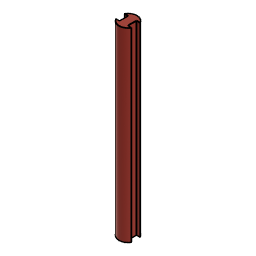
Osa krokoměru v6 (Autodesk Fusion 360 design; units mm, degrees)
Autodesk Fusion 360 part; units mm, degrees
sketch "Profil" plane through (0, 0, 0) normal (0, 0, 1) x (1, 0, 0)
  circle A0 centre (0, 0) radius 4.3
  line L0 (3.8066, -2) -> (-3.8066, -2)
  line L1 (-3.8066, -2) -> (-3.8066, 2)
  line L2 (-3.8066, 2) -> (3.8066, 2)
  line L3 (3.8066, 2) -> (3.8066, -2)
  line L4 (3.8066, -2) -> (-3.8066, 2) construction
  line L5 (-3.8066, -2) -> (3.8066, 2) construction
  line L6 (2, -2) -> (-2, -2)
  line L7 (-2, -2) -> (-2, 2)
  line L8 (-2, 2) -> (2, 2)
  line L9 (2, 2) -> (2, -2)
  line L10 (2, -2) -> (-2, 2) construction
  line L11 (-2, -2) -> (2, 2) construction
  line L12 (3.6946, 2.2) -> (3.6946, -2.2)
  dimension "d1" = 8.6
  dimension "d2" = 4
  dimension "d3" = 4
  dimension "d4" = 0.2
  constraint coincident A0.centre origin
  constraint horizontal L0
  constraint perpendicular L0 L1
  constraint parallel L0 L2
  constraint parallel L1 L3
  constraint coincident L4 A0.centre
  constraint coincident L5 A0.centre
  constraint coincident A0 L0.start
  constraint horizontal L6
  constraint perpendicular L6 L7
  constraint parallel L6 L8
  constraint parallel L7 L9
  constraint coincident L10 A0.centre
  constraint coincident L11 A0.centre
  constraint coincident L0 L6.start
  constraint coincident A0 L12.start
  constraint coincident A0 L12.end
  constraint perpendicular L0 L12
  measures "d1" diameter of A0
  measures "d2" distance of L0.start L2.end
  measures "d3" distance of L7 L9
  measures "d4" distance of L0 L12.end
extrude "Extrude1" add sketch "Profil" along normal blind 88.5 contours A0 L2 L8 L12 | A0 L0 L6 L12 | L0 L2 L6 L7 L8 L9
fillet "Fillet1" radius 0.1 2 edges at (-3.8066, 2, 44.25) (-3.8066, -2, 44.25)
chamfer "Chamfer1" distance 0.1 angle 45 4 edges at (-2, -2, 44.25) (-2, 2, 44.25) (2, -2, 44.25) (2, 2, 44.25)
chamfer "Chamfer2" distance 0.1 angle 45 2 faces at (0.6667, -0.6333, 88.5) (0.6667, -0.6333, 0)
named bodies: "Osa krokoměru"
